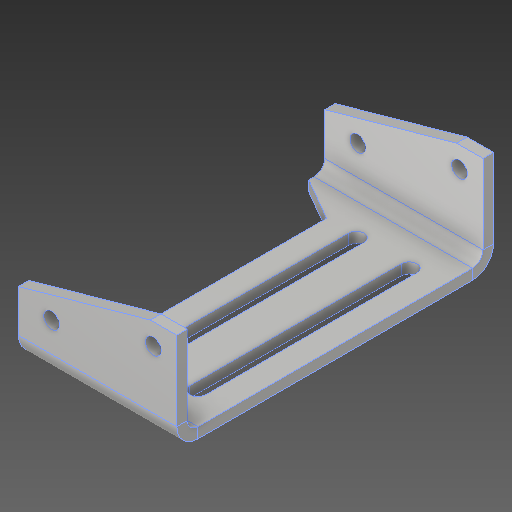
# Autodesk Inventor part: trackball_l
Saved by Autodesk Inventor 2018 (Build 220112000, 112)
## iProperties
Created: 2018-07-04
Part Number: trackball_l
Material: アルミニウム 6061
Document SubType Name: Sheet Metal
Designer: NaMACHAN
Mass: 10.3803 g
Surface Area: 47.5768 cm^2
Volume: 3.84456 cm^3
Density: 2.7 g/cm^3
Sheet Metal Rule: Default
Appearance: アルミニウム - フラット
Author: NaMACHAN
Autodesk Inventor part; units mm, degrees
ref_plane "YZ Plane" through (0, 0, 0) normal (1, 0, 0) x (0, 1, 0)
ref_plane "XZ Plane" through (0, 0, 0) normal (0, 1, 0) x (-1, 0, 0)
ref_plane "XY Plane" through (0, 0, 0) normal (0, 0, 1) x (1, 0, 0)
sketch "スケッチ1" plane through (0, 0, 0) normal (0, 1, 0) x (-1, 0, 0)
  line L0 (-15, -28) -> (15, -28)
  line L1 (15, 28) -> (-15, 28)
  line L2 (-15, 28) -> (-15, -28)
  line L3 (-15, -28) -> (15, 28) construction
  line L4 (15, -28) -> (-15, 28) construction
  line L5 (15, -28) -> (15, -25)
  line L6 (15, -25) -> (7, -20.3812)
  line L7 (7, -20.3812) -> (7, 20.3812)
  line L8 (7, 20.3812) -> (15, 25)
  line L9 (15, 25) -> (15, 28)
  point P0 (0, 0)
  dimension "d0" = 30
  dimension "d1" = 56
  dimension "d36" = 120
  dimension "d37" = 120
  dimension "d38" = 3
  dimension "d39" = 8
  dimension "d43" = 3
  measures "d0" distance of L1.end L1.start
  measures "d1" distance of L1.start L0.end
  measures "d36" angle of L5 L6
  measures "d37" angle of L9 L8
  measures "d38" distance of L1.start L8.end
  measures "d39" distance between parallel lines of L9 L7
  measures "d43" distance of L0.end L5.end
extrude "プレート1" add sketch "スケッチ1" along normal blind 2
sketch "スケッチ2" plane through (-15, 0, 28) normal (0, 0, 1) x (1, 0, 0)
  line L0 (0, 2) -> (30, 2)
  line L1 (0, 2) -> (0, 12)
  line L2 (0, 12) -> (25, 19)
  line L3 (25, 19) -> (30, 19)
  line L4 (30, 19) -> (30, 2)
  line L5 (0, 0) -> (0, 2)
  line L6 (30, 2) -> (0, 2)
  point P0 (15, 0)
  dimension "d3" = 10
  dimension "d4" = 5
  dimension "d5" = 17
  measures "d3" distance of L0.start L1.end
  measures "d4" distance of L2.end L3.end
  measures "d5" distance between parallel lines of L3 L0
sheet face with bend "面2" sketch "スケッチ2" thickness 2 toward (0, 0, 1) bend radius 2 relief tear relief width 2 relief depth 1
bend "曲げ1"
sketch "スケッチ3" plane through (15, 0, -28) normal (0, 0, -1) x (-1, 0, 0)
  line L0 (0, 0) -> (0, 2)
  line L1 (0, 2) -> (0, 19)
  line L2 (0, 19) -> (5, 19)
  line L3 (0, 19) -> (5, 19)
  line L4 (30, 12) -> (30, 4)
  line L5 (5, 19) -> (30, 12)
  line L6 (30, 0) -> (30, 2)
  line L7 (30, 12) -> (30, 2)
  line L8 (30, 2) -> (0, 2)
  point P0 (15, 0)
sheet face with bend "面3" sketch "スケッチ3" thickness 2 toward (0, 0, -1) bend radius 2 relief tear relief width 2 relief depth 1
bend "曲げ2"
sketch "スケッチ4" plane through (15, 0, -30) normal (0, 0, -1) x (-1, 0, 0)
  line L0 (5, 19) -> (30, 12) projected
  line L1 (0, 19) -> (5, 19) projected
  point P0 (15, 0)
  point P1 (4.4506, 15)
  point P2 (23.7098, 9.6074)
  dimension "d16" = 4
  dimension "d17" = 4
  dimension "d18" = 20
  dimension "d19" = 4
  measures "d16" distance from line of L0 point (23.71, 9.607)
  measures "d17" distance from line of L0 point (4.451, 15)
  measures "d18" distance of point (4.451, 15) point (23.71, 9.607)
  measures "d19" distance from line of L1 point (4.451, 15)
hole "穴1" at (10.5494, 15, -30) at (-8.7098, 9.6074, -30) direction (0, 0, 1) diameter 3 end through all
sketch "スケッチ5" plane through (0, 2, 0) normal (0, 1, 0) x (1, 0, 0)
  line L0 (10.5, 20) -> (10.5, -20)
  arc A0 (7.5, -20) -> (10.5, -20) centre (9, -20) ccw
  line L1 (7.5, -20) -> (7.5, 20)
  arc A1 (10.5, 20) -> (7.5, 20) centre (9, 20) ccw
  line L2 (0.5, 20) -> (0.5, -20)
  arc A2 (-2.5, -20) -> (0.5, -20) centre (-1, -20) ccw
  line L3 (-2.5, -20) -> (-2.5, 20)
  arc A3 (0.5, 20) -> (-2.5, 20) centre (-1, 20) ccw
  line L4 (15, 26) -> (15, -26) projected
  line L5 (15, 26) -> (-15, 26) projected
  line L6 (-15, -26) -> (15, -26) projected
  line L7 (-15, 25) -> (-15, 26) projected
  point P0 (0, 0)
  dimension "d27" = 6
  dimension "d30" = 1.5
  dimension "d31" = 1.5
  dimension "d32" = 6
  dimension "d33" = 6
  dimension "d41" = 14
  constraints: 8 end point, 8 point on circle, 6 tangent, 4 centre point, 4 horizontal alignment, 2 vertical, 1 parallel, 1 vertical alignment
  measures "d27" distance from line of L4 A1.centre
  measures "d30" radius of A3
  measures "d31" radius of A1
  measures "d32" distance from line of L5 A1.centre
  measures "d33" distance from line of L6 A0.centre
  measures "d41" distance from line of A3.centre L7
extrude "押し出し1" cut sketch "スケッチ5" against normal blind 10
equation "\"d25\" = Thickness"
equation "\"d2\" = Thickness"
equation "\"d6\" = BendRadius"
equation "\"d7\" = BendReliefWidth"
equation "\"d9\" = MinimumRemnant"
equation "\"d8\" = BendReliefDepth"
equation "\"d10\" = TransitionRadius"
equation "\"d11\" = BendRadius"
equation "\"d12\" = BendReliefWidth"
equation "\"d14\" = MinimumRemnant"
equation "\"d13\" = BendReliefDepth"
equation "\"d15\" = TransitionRadius"
equation "\"BendRadius\" = Thickness"
equation "\"BendReliefWidth\" = Thickness"
equation "\"BendReliefDepth\" = 0.5 * Thickness"
equation "\"CornerReliefSize\" = 4 * Thickness"
equation "\"MinimumRemnant\" = 2 * Thickness"
equation "\"TransitionRadius\" = BendRadius"
equation "\"JacobiRadiusSize\" = Thickness"
equation "\"GapSize\" = Thickness"
equation "\"Thickness\" = 2"
